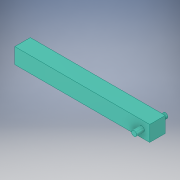
# Autodesk Inventor part: Arm
Saved by Autodesk Inventor 2018 (Build 220112000, 112)
## iProperties
Created: 2017-12-31
Part Number: Arm
Material: Generic
Document SubType Name: Modeling
Designer: suchanek
Density: 1 g/cm^3
Appearance: Default
Author: suchanek
Autodesk Inventor part; units mm, degrees
ref_plane "YZ Plane" through (0, 0, 0) normal (1, 0, 0) x (0, 1, 0)
ref_plane "XZ Plane" through (0, 0, 0) normal (0, 1, 0) x (-1, 0, 0)
ref_plane "XY Plane" through (0, 0, 0) normal (0, 0, 1) x (1, 0, 0)
sketch "Sketch1" plane through (0, 0, 0) normal (0, 0, 1) x (1, 0, 0)
  line L0 (0, 6) -> (52, 6)
  line L1 (56, 0) -> (0, 0)
  line L2 (52, 0) -> (52, 6)
  circle A0 centre (49, 3) radius 1
  line L3 (0, 0) -> (0, 6)
  dimension "d26" = 2
  dimension "d29" = 52
  dimension "d30" = 3
  dimension "d31" = 3
  dimension "d32" = 6
  constraints: 8 end point, 5 point on line, 1 centre point, 1 horizontal, 1 parallel, 1 perpendicular
  measures "d26" diameter of A0
  measures "d29" distance between parallel lines of L3 L2
  measures "d30" distance from line of L2 A0.centre
  measures "d31" distance from line of L0 A0.centre
  measures "d32" distance between parallel lines of L0 L1
extrude "Extrusion1" add sketch "Sketch1" along normal mid plane 6 contours L0 L2 L1 L3 | A0
sketch "Sketch6" plane through (0, 0, 3) normal (0, 0, 1) x (1, 0, 0)
  line L0 (0, 6) -> (52, 6)
  line L1 (56, 0) -> (0, 0)
  line L2 (52, 0) -> (52, 6)
  circle A0 centre (49, 3) radius 1
  line L3 (0, 0) -> (0, 6)
  dimension "d34" = 2
  dimension "d35" = 52
  dimension "d36" = 3
  dimension "d37" = 3
  dimension "d38" = 6
  constraints: 8 end point, 5 point on line, 1 centre point, 1 horizontal, 1 parallel, 1 perpendicular
  measures "d34" diameter of A0
  measures "d35" distance between parallel lines of L3 L2
  measures "d36" distance from line of L2 A0.centre
  measures "d37" distance from line of L0 A0.centre
  measures "d38" distance between parallel lines of L0 L1
extrude "Extrusion4" add sketch "Sketch6" along normal blind 3 and the other way blind 9 contours A0
body "Solid1"
